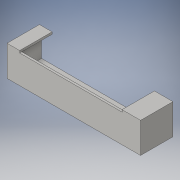
# Autodesk Inventor part: cradle
Saved by Autodesk Inventor 2016 SP1 (Build 200210100, 210)
## iProperties
Created: 2016-05-02
Part Number: cradle
Material: Generic
Document SubType Name: Modeling
Designer: Wes
Density: 1 g/cm^3
Appearance: Default
Author: Wes
Autodesk Inventor part; units mm, degrees
ref_plane "YZ Plane" through (0, 0, 0) normal (1, 0, 0) x (0, 1, 0)
ref_plane "XZ Plane" through (0, 0, 0) normal (0, 1, 0) x (-1, 0, 0)
ref_plane "XY Plane" through (0, 0, 0) normal (0, 0, 1) x (1, 0, 0)
sketch "Sketch1" plane through (0, 0, 0) normal (0, 0, 1) x (1, 0, 0)
  line L0 (-77.47, 15.6845) -> (77.47, 15.6845)
  line L1 (77.47, 15.6845) -> (77.47, -15.6845)
  line L2 (77.47, -15.6845) -> (-77.47, -15.6845)
  line L3 (-77.47, -15.6845) -> (-77.47, 15.6845)
  line L4 (-80.01, 18.2372) -> (80.01, 18.2372)
  line L5 (80.01, 18.2372) -> (80.01, -18.2118)
  line L6 (80.01, -18.2118) -> (-80.01, -18.2118)
  line L7 (-80.01, -18.2118) -> (-80.01, 18.2372)
  line L8 (-64.8716, 15.6845) -> (-64.8716, 18.2372)
  line L9 (57.7977, 15.6845) -> (57.7977, 18.2372)
  point P0 (0, 0)
  dimension "d0" = 154.94
  dimension "d1" = 31.369
  dimension "d2" = 160.02
  dimension "d3" = 36.449
  constraints: 20 end point, 4 parallel, 4 perpendicular, 4 point on line, 2 horizontal
  measures "d0" distance of L1.end L2.end
  measures "d1" distance of L0.end L1.end
  measures "d2" distance of L5.end L6.end
  measures "d3" distance of L4.end L5.end
extrude "front" add sketch "Sketch1" along normal blind 2.54 contours L0 L1 L2 L3
extrude "sides" add sketch "Sketch1" along normal blind 2.54 and the other way blind 36.2966 contours L3 L2 L1 L0 L9 L4 L5 L6 L7 L8
body "Solid1"
